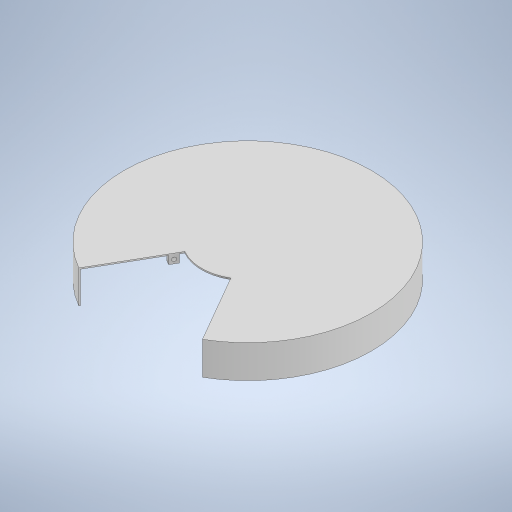
# Autodesk Inventor part: Cover
Saved by Autodesk Inventor 2024 (Build 280153000, 153)
## iProperties
Created: 2023-12-19
Part Number: Cover
Material: Generic
Document SubType Name: Modeling
Designer: 96279
Density: 1 g/cm^3
Appearance: Default
Author: 96279
Autodesk Inventor part; units mm, degrees
ref_plane "YZ Plane" through (0, 0, 0) normal (1, 0, 0) x (0, 1, 0)
ref_plane "XZ Plane" through (0, 0, 0) normal (0, 1, 0) x (-1, 0, 0)
ref_plane "XY Plane" through (0, 0, 0) normal (0, 0, 1) x (1, 0, 0)
sketch "Sketch1" plane through (0, 0, 0) normal (0, 1, 0) x (-1, 0, 0)
  circle A0 centre (0, 0) radius 94
  dimension "d0" = 188
  constraints: 1 centre point, 1 coincident
  measures "d0" diameter of A0
extrude "Extrusion1" add sketch "Sketch1" along normal blind 25
sketch "Sketch2" plane through (0, 0, 0) normal (0, -1, 0) x (1, 0, 0)
  point P0 (0, 0)
  point P1 (0, 0)
  constraints: 1 coincident
hole "Hole1" at (0, 0, 0) direction (0, 1, 0) diameter 186 depth 24
sketch "Sketch11" plane through (0, 25, 0) normal (0, 1, 0) x (1, 0, 0)
  circle A0 centre (0, 0) radius 94.1047
  circle A1 centre (0, 0) radius 35
  line L0 (35, 0) -> (94.1047, 0)
  line L1 (17.5, 30.3109) -> (47.0523, 81.4971)
  line L2 (-17.5, 30.3109) -> (-47.0523, 81.4971)
  line L3 (-35, 0) -> (-94.1047, 0)
  line L4 (-17.5, -30.3109) -> (-47.0523, -81.4971)
  line L5 (17.5, -30.3109) -> (47.0523, -81.4971)
  dimension "d46" = 70
  dimension "d49" = 360
  constraints: 12 end point, 2 coincident, 1 horizontal, 25 other
extrude "Extrusion4" cut sketch "Sketch11" against normal blind 30 contours A0 L4 A1 L5
sketch "Sketch5" plane through (0, 24, 0) normal (0, -1, 0) x (1, 0, 0)
  circle A0 centre (0.0185, 0.5394) radius 32.5
  circle A1 centre (0.0185, 0.5394) radius 91
  line L0 (0.0185, -31.9606) -> (0.0185, -90.4606)
  line L1 (-28.1273, -15.7106) -> (-78.7898, -44.9606)
  line L2 (-28.1273, 16.7894) -> (-78.7898, 46.0394)
  line L3 (0.0185, 33.0394) -> (0.0185, 91.5394)
  line L4 (28.1643, 16.7894) -> (78.8268, 46.0394)
  line L5 (27.2527, -15.1843) -> (78.8268, -44.9606)
  line L6 (30.5108, -13.5333) -> (27.5108, -18.7294)
  line L7 (27.5108, -18.7294) -> (31.8409, -21.2294)
  line L8 (31.8409, -21.2294) -> (34.8409, -16.0333)
  line L9 (34.8409, -16.0333) -> (30.5108, -13.5333)
  line L10 (-2.9302, -37.8595) -> (3.0698, -37.8595)
  line L11 (3.0698, -32.8595) -> (-2.9302, -32.8595)
  line L12 (-2.9302, -32.8595) -> (-2.9302, -37.8595)
  line L13 (3.0698, -37.8595) -> (3.0698, -32.8595)
  point P0 (0, 0)
  point P1 (24.0416, -20.6125)
  point P2 (3.0698, -35.3595)
  dimension "d23" = 65
  dimension "d30" = 360
  dimension "d38" = 6
  dimension "d39" = 5
  dimension "d40" = 6
  dimension "d41" = 5
  constraints: 28 end point, 4 parallel, 2 coincident, 2 perpendicular, 2 vertical alignment, 1 midpoint, 1 vertical, 21 other
  measures "d38" distance of L8.start L8.end
  measures "d39" distance of L8.end L6.start
  measures "d40" distance of L13.end L11.end
  measures "d41" distance of L11.end L12.end
extrude "Extrusion3" add sketch "Sketch5" along normal blind 0.1 contours L6 L9 L8 L5 | L5 L8 L7 L6 | L11 L13 L10 L0 | L0 L10 L12 L11
sketch "Sketch12" plane through (-47, 0, 81.4064) normal (0.8660254, 0, 0.5) x (0.5, 0, -0.8660254)
  point P0 (94, 0)
sketch "Sketch13" plane through (-47, 0, 81.4064) normal (0.8660254, 0, 0.5) x (0.5, 0, -0.8660254)
  line L0 (59, 24) -> (1, 24) projected
  line L1 (50, 24) -> (56, 24)
  line L2 (56, 24) -> (56, 18)
  line L3 (56, 18) -> (50, 18)
  line L4 (50, 18) -> (50, 24)
  line L5 (59, 25) -> (59, 24) projected
  point P0 (94, 0)
  dimension "d53" = 6
  dimension "d54" = 6
  dimension "d55" = 3
  constraints: 8 end point, 2 parallel, 1 horizontal, 1 perpendicular, 1 point on line
  measures "d53" distance of L3.end L1.start
  measures "d54" distance of L2.end L3.end
  measures "d55" distance between parallel lines of L2 L5
extrude "Extrusion5" add sketch "Sketch13" against normal blind 3.5
sketch "Sketch14" plane through (-47, 0, 81.4064) normal (0.8660254, 0, 0.5) x (0.5, 0, -0.8660254)
  circle A0 centre (53, 21) radius 1.5
  line L0 (50, 24) -> (50, 18) projected
  line L1 (50, 18) -> (56, 18) projected
  point P0 (94, 0)
  dimension "d58" = 3
  dimension "d59" = 3
  dimension "d60" = 3
  constraints: 1 centre point
  measures "d58" diameter of A0
  measures "d59" distance from line of L0 A0.centre
  measures "d60" distance from line of L1 A0.centre
hole "Hole2" at (-20.5, 21, 35.507) direction (-0.8660254, 0, -0.5) diameter 3 depth 29
sketch "Sketch15" plane through (47, 0, 81.4064) normal (-0.8660254, 0, 0.5) x (0.5, 0, 0.8660254)
  line L0 (-56, 24) -> (-50, 24)
  line L1 (-50, 24) -> (-50, 18)
  line L2 (-50, 18) -> (-56, 18)
  line L3 (-56, 18) -> (-56, 24)
  line L4 (-59, 25) -> (-59, 24) projected
  line L5 (-1, 24) -> (-59, 24) projected
  point P0 (-94, 0)
  dimension "d68" = 6
  dimension "d69" = 6
  dimension "d70" = 3
  dimension "d71" = 0
  constraints: 8 end point, 2 parallel, 1 horizontal, 1 perpendicular
  measures "d68" distance of L0.end L1.end
  measures "d69" distance of L1.end L2.end
  measures "d70" distance between parallel lines of L4 L3
  measures "d71" distance between parallel lines of L5 L0
extrude "Extrusion6" add sketch "Sketch15" against normal blind 3.5
sketch "Sketch16" plane through (47, 0, 81.4064) normal (-0.8660254, 0, 0.5) x (0.5, 0, 0.8660254)
  circle A0 centre (-53, 21) radius 1.5
  line L0 (-56, 24) -> (-56, 18) projected
  line L1 (-50, 24) -> (-56, 24) projected
  point P0 (-94, 0)
  dimension "d74" = 3
  dimension "d75" = 3
  dimension "d76" = 3
  constraints: 1 centre point
  measures "d74" diameter of A0
  measures "d75" distance from line of L0 A0.centre
  measures "d76" distance from line of L1 A0.centre
hole "Hole3" at (20.5, 21, 35.507) direction (0.8660254, 0, -0.5) diameter 3 depth 29
body "Solid1"
